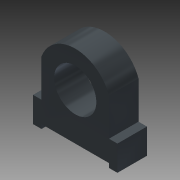
# Autodesk Inventor part: HW 4 Part 5
Saved by Autodesk Inventor 2015 SP1 (Build 190203100, 203)
## iProperties
Created: 2016-01-25
Part Number: HW 4 Part 5
Material: Iron, Cast
Document SubType Name: Modeling
Designer: melissa.roth
Density: 7.15 g/cm^3
Appearance: Iron Gray
Mass: 2986.25 g
Surface Area: 492.772 cm^2
Volume: 417.657 cm^3
Author: melissa.roth
Autodesk Inventor part; units mm, degrees
ref_plane "YZ Plane" through (0, 0, 0) normal (1, 0, 0) x (0, 1, 0)
ref_plane "XZ Plane" through (0, 0, 0) normal (0, 1, 0) x (-1, 0, 0)
ref_plane "XY Plane" through (0, 0, 0) normal (0, 0, 1) x (1, 0, 0)
sketch "Sketch1" plane through (0, 0, 0) normal (0, 0, 1) x (1, 0, 0)
  line L0 (0, 0) -> (12.7, 0)
  line L1 (12.7, 0) -> (12.7, 6.35)
  line L2 (12.7, 6.35) -> (114.3, 6.35)
  line L3 (114.3, 6.35) -> (114.3, 0)
  line L4 (114.3, 0) -> (127, 0)
  line L5 (127, 0) -> (127, 38.1)
  line L6 (127, 38.1) -> (114.3, 38.1)
  line L7 (114.3, 38.1) -> (114.3, 47.625)
  line L8 (12.7, 47.625) -> (12.7, 38.1)
  line L9 (12.7, 38.1) -> (0, 38.1)
  line L10 (0, 38.1) -> (0, 0)
  circle A0 centre (63.5, 76.2) radius 31.75
  line L11 (12.7, 47.625) -> (12.7, 94.439)
  line L12 (114.3, 47.625) -> (114.3, 94.439)
  arc A1 (114.3, 94.439) -> (12.7, 94.439) centre (63.5, 76.2) ccw
  dimension "d0" = 38.1
  dimension "d1" = 101.6
  dimension "d2" = 12.7
  dimension "d3" = 6.35
  dimension "d4" = 63.5
  dimension "d5" = 76.2
  dimension "d6" = 63.5
  constraints: 26 end point, 6 point on line, 5 perpendicular, 3 equal length, 2 centre point, 2 point on circle, 1 coincident, 1 horizontal, 1 vertical
  measures "d0" distance of L9.end L0.start
  measures "d1" distance of L1.end L2.end
  measures "d2" distance of L3.end L4.end
  measures "d3" distance of L2.end L3.end
  measures "d4" diameter of A0
  measures "d5" vertical distance of A0.centre L0.start
  measures "d6" distance from line of A0.centre L10
extrude "Extrusion1" add sketch "Sketch1" along normal blind 44.45
body "Solid1"
